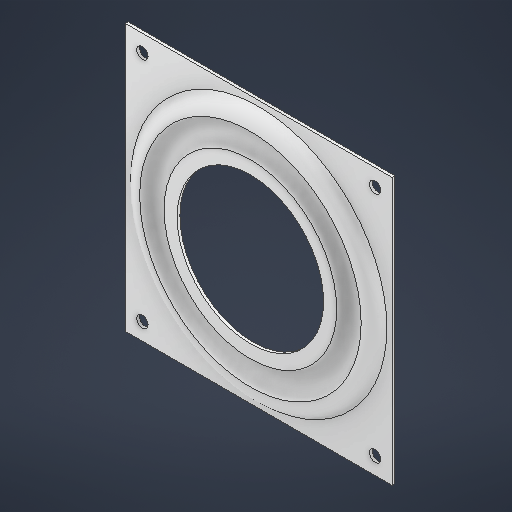
# Autodesk Inventor part: plataforma_giratória_94L)4polegadas)
Saved by Autodesk Inventor 2025.2 (Build 292293000, 293)
## iProperties
Created: 2025-04-27
Part Number: plataforma_giratória_94L)4polegadas)
Material: Generic
Document SubType Name: Modeling
Designer: Tiago
Density: 1 g/cm^3
Appearance: Default
Author: Tiago
Autodesk Inventor part; units mm, degrees
ref_plane "YZ Plane" through (0, 0, 0) normal (1, 0, 0) x (0, 1, 0)
ref_plane "XZ Plane" through (0, 0, 0) normal (0, 1, 0) x (-1, 0, 0)
ref_plane "XY Plane" through (0, 0, 0) normal (0, 0, 1) x (1, 0, 0)
sketch "Sketch1" plane through (0, 0, 0) normal (0, 0, 1) x (1, 0, 0)
  circle A0 centre (0, 0) radius 17.5
  line L0 (-47, 47) -> (47, 47)
  line L1 (47, 47) -> (47, -47)
  line L2 (47, -47) -> (-47, -47)
  line L3 (-47, -47) -> (-47, 47)
  line L4 (-47, 47) -> (47, -47) construction
  line L5 (47, 47) -> (-47, -47) construction
  line L6 (0, 41) -> (0, -41) construction
  line L7 (0, 41) -> (41, 41) construction
  line L8 (-41, 0) -> (41, 0) construction
  circle A1 centre (41, 41) radius 2
  circle A2 centre (41, -41) radius 2
  circle A3 centre (-41, 41) radius 2
  circle A4 centre (-41, -41) radius 2
  circle A5 centre (0, 0) radius 41
  circle A6 centre (0, 0) radius 42.925
  dimension "di" = 35
  dimension "L" = 94
  dimension "d2" = 94
  dimension "d4" = 82
  dimension "d5" = 82
  dimension "d6" = 4
  dimension "d20" = 85.85
  constraints: 18 end point, 6 centre point, 4 coincident, 4 midpoint, 3 symmetric about line, 2 horizontal, 2 parallel, 2 perpendicular, 1 point on line, 1 vertical alignment, 5 other
  measures "di" diameter of A0
  measures "L" distance of L1.end L2.end
  measures "d2" distance of L0.end L1.end
  measures "d4" distance of L6.start L6.end
  measures "d5" distance of L8.start L8.end
  measures "d6" diameter of A1
  measures "d20" diameter of A6
extrude "Extrusion2" add sketch "Sketch1" along normal blind 1 contours L0 L1 L2 L3
sketch "Sketch2" plane through (0, 0, 0) normal (0, 1, 0) x (-1, 0, 0)
  line L0 (42.925, 1) -> (47, 1) projected
  line L1 (47, 1) -> (47, 0) projected
  line L2 (-47, 0) -> (-47, 1) projected
  line L3 (-47, 1) -> (-42.925, 1) projected
  line L4 (47, 0) -> (44.65, 0)
  line L5 (-47, 0) -> (47, 0) projected
  line L6 (44.65, 0) -> (39.65, 0)
  line L7 (39.65, 0) -> (39.65, 3) construction
  arc A0 (44.65, 0) -> (39.65, 3) centre (39.452, -2.9967) ccw
  line L8 (39.65, 3) -> (29.8, 3) construction
  arc A1 (29.8, 3) -> (39.65, 3) centre (34.725, 5.5426) ccw
  line L9 (29.8, 3) -> (25.8, 3)
  arc A2 (45.735, -0.0258) -> (39.0291, 3.9404) centre (39.452, -2.9967) ccw
  arc A3 (30.4174, 3.95) -> (39.0291, 3.9404) centre (34.725, 5.5426) ccw
  line L10 (30.4174, 3.95) -> (25.8, 3.95)
  line L11 (-47, 1) -> (47, 1) projected
  line L12 (43.927, 1) -> (45.1378, 1)
  line L13 (25.8, 3.95) -> (25.8, 3)
  line L14 (47, 0) -> (42.925, 0) projected
  line L15 (-42.925, 0) -> (-47, 0) projected
  line L16 (0, -4.8295) -> (0, 8.0307) projected
  line L17 (42.925, 0) -> (42.925, 1) projected
  line L18 (-42.925, 1) -> (-42.925, 0) projected
  line L19 (23.595, 4) -> (45.4292, 4)
  point P0 (0, 0)
  point P1 (43.927, 1)
  dimension "d11" = 2.35
  dimension "d12" = 5
  dimension "d13" = 3
  dimension "d14" = 6
  dimension "d15" = 9.85
  dimension "d16" = 4
  dimension "d17" = 0.95
  constraints: 18 end point, 10 point on circle, 4 centre point, 4 point on line, 3 horizontal, 1 perpendicular, 1 tangent, 1 vertical, 2 other
  measures "d11" distance of L1.end L4.end
  measures "d12" distance of L4.end L6.end
  measures "d13" distance of L6.end L7.end
  measures "d14" radius of A0
  measures "d15" distance of L7.end L8.end
  measures "d16" distance of L8.end L9.end
  measures "d17" radial gap between concentric circles of A0 A2
revolve "Revolution1" add sketch "Sketch2" angle 360 about axis through (0, 0, -10) along (0, 0, 1) contours A0 A1 L11 A3 A2 L0 | A1 L11 A3 | A1 L9 L13 L10 A3 L11
fillet "Fillet2" radius 1 1 edges at (-42.925, 0, 0) curvature continuous yes
equation "\"d2\" = L"
equation "\"d4\" = L_furos"
equation "\"d5\" = L_furos"
equation "\"L_furos\" = 82"
body "Solid1"
